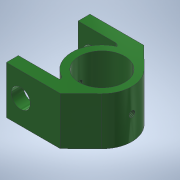
# Autodesk Inventor part: MANCAL_SUPORTE_EIXO
Saved by Autodesk Inventor 2020 (Build 240168000, 168)
## iProperties
Created: 2016-02-21
Part Number: MANCAL_SUPORTE_EIXO
Material: SAE 1010/1020
Document SubType Name: Modeling
Designer: Everton
Authority: Rafael Salvador
Manufacturer: Standard
Standards Organization: Custom
Density: 7.86 g/cm^3
Appearance: Steel
Manager: Standard
Author: Everton
Comments: -
Revision Number: 00
Autodesk Inventor part; units mm, degrees
ref_plane "YZ Plane" through (0, 0, 0) normal (1, 0, 0) x (0, 1, 0)
ref_plane "XZ Plane" through (0, 0, 0) normal (0, 1, 0) x (-1, 0, 0)
ref_plane "XY Plane" through (0, 0, 0) normal (0, 0, 1) x (1, 0, 0)
sketch "Sketch1" plane through (0, 0, 0) normal (0, 0, 1) x (1, 0, 0)
  circle A0 centre (36.1481, 50.2593) radius 25
  circle A1 centre (36.1481, 50.2593) radius 19
  line L0 (36.1481, 75.2593) -> (1.1481, 75.2593)
  line L1 (36.1481, 85.2593) -> (-8.8519, 85.2593)
  line L2 (-8.8519, 85.2593) -> (-8.8519, 75.2593)
  line L3 (36.1481, 85.2593) -> (36.1481, 75.2593)
  line L4 (1.1481, 75.2593) -> (-8.8519, 75.2593)
  line L5 (36.1481, 25.2593) -> (1.1481, 25.2593)
  line L6 (36.1481, 15.2593) -> (-8.8519, 15.2593)
  line L7 (1.1481, 25.2593) -> (-8.8519, 25.2593)
  line L8 (36.1481, 15.2593) -> (36.1481, 25.2593)
  line L9 (-8.8519, 15.2593) -> (-8.8519, 25.2593)
  line L10 (36.1481, 85.2593) -> (53.6445, 68.1164)
  line L11 (36.1481, 15.2593) -> (53.6445, 32.4021)
  arc A2 (25.8947, 73.0598) -> (22.1511, 75.2593) centre (22.1511, 70.9735) ccw
  arc A3 (25.8027, 25.2593) -> (23.935, 28.4455) centre (22.1511, 25.2593) ccw
  point P0 (0, 0)
  dimension "d0" = 38
  dimension "d1" = 10
  constraints: 24 end point, 9 point on circle, 4 centre point, 4 tangent, 3 point on line, 1 coincident, 1 perpendicular, 1 vertical
  measures "d0" diameter of A1
  measures "d1" distance between parallel lines of L0 L1
extrude "Extrusion1" add sketch "Sketch1" along normal blind 40
sketch "Sketch2" plane through (-8.8519, 15.2593, 0) normal (0, -1, 0) x (1, 0, 0)
  line L0 (0, 0) -> (0, 40) projected
  line L1 (0, 20) -> (12, 20)
  circle A0 centre (12, 20) radius 8
  point P0 (8.8519, 0)
  dimension "d4" = 12
  dimension "d5" = 16
  constraints: 2 end point, 1 centre point, 1 coincident, 1 horizontal, 1 midpoint
  measures "d4" distance of L1.start L1.end
  measures "d5" diameter of A0
extrude "Extrusion2" cut sketch "Sketch2" against normal blind 80
sketch "Sketch4" plane through (0, 0, 0) normal (1, 0, 0) x (0, 1, 0)
  line L0 (15.2593, 0) -> (15.2593, 40) projected
  line L1 (15.2593, 20) -> (85.6982, 20)
  point P0 (0, 0)
  point P1 (50.4787, 20)
  constraints: 2 end point, 2 midpoint, 1 horizontal
hole "Hole1" at (0, 50.4787, 20) direction (1, 0, 0) diameter 4.917 depth 85.1 tip angle 118 thread size "M6x1" class "6H" standard "ANSI Metric M Profile"
body "Solid1"
